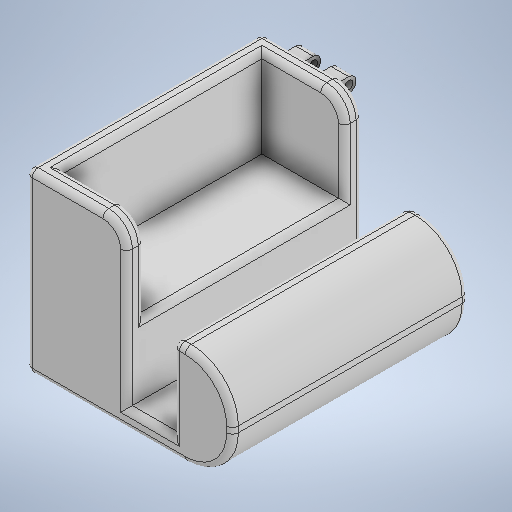
# Autodesk Inventor part: scrambler_chariot
Saved by Autodesk Inventor 2025.2 (Build 292293000, 293)
## iProperties
Created: 2025-10-10
Part Number: scrambler_chariot
Material: Generic
Document SubType Name: Modeling
Designer: pascu
Density: 1 g/cm^3
Appearance: Default
Mass: 35.9125 g
Surface Area: 129.419 cm^2
Volume: 35.9125 cm^3
Author: pascu
Autodesk Inventor part; units mm, degrees
ref_plane "YZ Plane" through (0, 0, 0) normal (1, 0, 0) x (0, 1, 0)
ref_plane "XZ Plane" through (0, 0, 0) normal (0, 1, 0) x (-1, 0, 0)
sketch "Sketch1" plane through (0, 0, 0) normal (0, 1, 0) x (-1, 0, 0)
  line L0 (0, 0) -> (-44.45, 0)
  line L1 (-44.45, 0) -> (-44.45, -50.8)
  line L2 (-44.45, -50.8) -> (0, -50.8)
  line L3 (0, -50.8) -> (0, 0)
  dimension "d0" = 44.45
  dimension "d1" = 50.8
  constraints: 8 end point, 2 parallel, 1 horizontal, 1 perpendicular
  measures "d0" distance of L2.end L1.end
  measures "d1" distance of L1.end L0.end
extrude "Extrusion1" add sketch "Sketch1" along normal blind 38.1
sketch "Sketch2" plane through (0, 38.1, 0) normal (0, 1, 0) x (1, 0, 0)
  line L0 (3.81, 3.81) -> (21.59, 3.81)
  line L1 (21.59, 3.81) -> (21.59, 46.99)
  line L2 (21.59, 46.99) -> (3.81, 46.99)
  line L3 (3.81, 46.99) -> (3.81, 3.81)
  line L4 (44.45, 50.8) -> (0, 50.8) projected
  line L5 (0, 50.8) -> (0, 0) projected
  line L6 (0, 0) -> (44.45, 0) projected
  dimension "d4" = 3.81
  dimension "d5" = 3.81
  dimension "d6" = 3.81
  dimension "d7" = 21.59
  constraints: 8 end point, 2 parallel, 1 horizontal, 1 perpendicular
  measures "d4" distance between parallel lines of L4 L2
  measures "d5" distance between parallel lines of L5 L3
  measures "d6" distance between parallel lines of L6 L0
  measures "d7" distance between parallel lines of L5 L1
extrude "Extrusion2" cut sketch "Sketch2" against normal blind 19.05
sketch "Sketch3" plane through (0, 38.1, 0) normal (0, 1, 0) x (1, 0, 0)
  line L0 (21.59, 46.99) -> (21.59, 3.81) projected
  line L1 (21.59, 0) -> (31.75, 0)
  line L2 (31.75, 0) -> (31.75, 50.8)
  line L3 (31.75, 50.8) -> (21.59, 50.8)
  line L4 (44.45, 50.8) -> (0, 50.8) projected
  line L5 (0, 0) -> (44.45, 0) projected
  line L6 (21.59, 50.8) -> (21.59, 0)
  dimension "d10" = 10.16
  constraints: 8 end point, 2 collinear, 1 horizontal, 1 parallel, 1 perpendicular, 1 vertical
  measures "d10" distance of L3.end L2.end
extrude "Extrusion3" cut sketch "Sketch3" against normal blind 34.29
sketch "Sketch4" plane through (0, 38.1, 0) normal (0, 1, 0) x (1, 0, 0)
  line L0 (44.45, 50.8) -> (31.75, 50.8) projected
  line L1 (44.45, 0) -> (44.45, 50.8) projected
  line L2 (31.75, 50.8) -> (31.75, 0) projected
  line L3 (31.75, 0) -> (44.45, 0) projected
  point P0 (0, 0)
extrude "Extrusion4" cut sketch "Sketch4" against normal blind 16.51
fillet "Fillet1" radius 10.16 2 edges at (44.45, 21.59, -25.4) (44.45, 0, -25.4)
ref_plane "Work Plane1" through (0, 0, -3.81) normal (0, 0, 1) x (1, 0, 0)
sketch "Sketch5" plane through (0, 0, -3.81) normal (0, 0, 1) x (1, 0, 0)
  arc A0 (44.45, 11.43) -> (34.29, 21.59) centre (34.29, 11.43) ccw projected
  arc A1 (34.29, 0) -> (44.45, 10.16) centre (34.29, 10.16) ccw projected
  line L0 (44.45, 10.16) -> (44.45, 11.43) projected
  arc A2 (40.64, 11.43) -> (34.29, 17.78) centre (34.29, 11.43) ccw
  line L1 (40.64, 11.43) -> (40.64, 10.16)
  arc A3 (34.29, 3.81) -> (40.64, 10.16) centre (34.29, 10.16) ccw
  line L2 (34.29, 17.78) -> (31.75, 17.78)
  line L3 (31.75, 3.81) -> (31.75, 21.59) projected
  line L4 (34.29, 3.81) -> (31.75, 3.81)
  line L5 (31.75, 3.81) -> (31.75, 17.78)
  point P0 (0, 0)
  dimension "d17" = 3.81
  constraints: 8 end point, 4 point on circle, 2 centre point, 2 horizontal, 1 collinear, 1 point on line, 2 other
  measures "d17" radial gap between concentric circles of A0 A2
extrude "Extrusion5" cut sketch "Sketch5" against normal blind 43.18
fillet "Fillet2" radius 5.08 2 edges at (21.59, 38.1, -1.905) (21.59, 38.1, -48.895)
fillet "Fillet3" radius 1.27 16 edges at (0, 38.1, -25.4) (3.81, 38.1, -25.4) (21.59, 19.05, -25.4) (0, 19.05, 0) (41.4742, 2.9758, 0) (44.45, 10.795, 0) (41.4742, 18.6142, 0) (33.02, 21.59, 0) (17.145, 0, 0) (41.4742, 18.6142, -50.8) (33.02, 21.59, -50.8) (41.4742, 2.9758, -50.8) (17.145, 0, -50.8) (44.45, 10.795, -50.8) (0, 19.05, -50.8) (0, 0, -25.4)
fillet "Fillet4" radius 1.27 18 edges at (20.1021, 36.6121, -50.8) (8.89, 38.1, -50.8) (0.372, 37.728, -50.428) (21.59, 18.415, -50.8) (20.1021, 36.6121, -46.99) (10.16, 38.1, -46.99) (3.175, 38.1, -46.99) (21.59, 18.415, -46.99) (21.59, 26.035, -46.99) (20.1021, 36.6121, -3.81) (10.16, 38.1, -3.81) (3.175, 38.1, -3.81) (21.59, 18.415, -3.81) (21.59, 26.035, -3.81) (20.1021, 36.6121, 0) (8.89, 38.1, 0) (0.372, 37.728, -0.372) (21.59, 18.415, 0)
fillet "Fillet5" radius 1.27 2 edges at (26.035, 3.81, -50.8) (26.035, 3.81, 0)
fillet "Fillet6" radius 1.27 7 edges at (31.75, 21.218, -50.428) (31.75, 21.59, -25.4) (31.75, 21.218, -0.372) (31.75, 12.065, 0) (31.75, 3.175, 0) (31.75, 12.065, -50.8) (31.75, 3.175, -50.8)
sketch "Sketch6" plane through (34.29, 1.27, -50.8) normal (0, 0, -1) x (-1, 0, 0)
  line L0 (33.02, 0) -> (0, 0) projected
  line L1 (13.9788, 0) -> (25.4088, 0)
  line L2 (25.4088, 0) -> (25.4088, 3.175)
  line L3 (25.4088, 3.175) -> (13.9788, 3.175)
  line L4 (13.9788, 3.175) -> (13.9788, 0)
  arc A0 (17.78, 35.56) -> (13.97, 31.75) centre (17.78, 31.75) ccw projected
  line L5 (17.78, 35.56) -> (29.21, 35.56)
  line L6 (29.21, 35.56) -> (29.21, 32.385)
  line L7 (29.21, 32.385) -> (17.78, 32.385)
  line L8 (17.78, 32.385) -> (17.78, 35.56)
  point P0 (34.29, -1.27)
  point P1 (25.4088, 0)
  dimension "d25" = 11.43
  dimension "d26" = 3.175
  dimension "d27" = 11.43
  dimension "d28" = 3.175
  constraints: 16 end point, 4 parallel, 2 horizontal, 2 perpendicular, 1 point on line
  measures "d25" distance of L3.end L2.end
  measures "d26" distance of L2.end L1.end
  measures "d27" distance of L6.end L7.end
  measures "d28" distance of L5.end L6.end
extrude "Extrusion6" add sketch "Sketch6" along normal blind 3.81
sketch "Sketch7" plane through (34.29, 1.27, -54.61) normal (0, 0, -1) x (-1, 0, 0)
  line L0 (29.21, 32.385) -> (17.78, 32.385) projected
  line L1 (21.59, 32.385) -> (25.4, 32.385)
  line L2 (25.4, 32.385) -> (25.4, 35.56)
  line L3 (25.4, 35.56) -> (21.59, 35.56)
  line L4 (21.59, 35.56) -> (21.59, 32.385)
  line L5 (29.21, 32.385) -> (29.21, 35.56) projected
  line L6 (17.78, 35.56) -> (17.78, 32.385) projected
  line L7 (13.9788, 3.175) -> (13.9788, 0) projected
  line L8 (13.9788, 0) -> (25.4088, 0) projected
  line L9 (17.7888, 0) -> (21.5988, 0)
  line L10 (21.5988, 0) -> (21.5988, 3.175)
  line L11 (21.5988, 3.175) -> (17.7888, 3.175)
  line L12 (17.7888, 3.175) -> (17.7888, 0)
  line L13 (25.4088, 0) -> (25.4088, 3.175) projected
  line L14 (25.4088, 3.175) -> (13.9788, 3.175) projected
  point P0 (34.29, -1.27)
  dimension "d31" = 3.175
  dimension "d32" = 3.81
  dimension "d33" = 3.81
  dimension "d34" = 3.175
  dimension "d35" = 3.81
  dimension "d36" = 3.81
  constraints: 16 end point, 4 parallel, 2 horizontal, 2 perpendicular, 1 collinear, 1 point on line
  measures "d31" distance of L1.end L2.end
  measures "d32" distance between parallel lines of L5 L2
  measures "d33" distance between parallel lines of L6 L4
  measures "d34" distance of L9.end L10.end
  measures "d35" distance between parallel lines of L7 L12
  measures "d36" distance between parallel lines of L13 L10
extrude "Extrusion7" cut sketch "Sketch7" against normal blind 3.81 contours L0 L4 L3 L2 | L11 L10 L8 L12
fillet "Fillet7" radius 1.5875 8 edges at (18.4062, 4.445, -54.61) (18.4062, 1.27, -54.61) (10.7862, 4.445, -54.61) (10.7862, 1.27, -54.61) (14.605, 33.655, -54.61) (14.605, 36.83, -54.61) (6.985, 33.655, -54.61) (6.985, 36.83, -54.61)
sketch "Sketch8" plane through (16.51, 33.655, -50.8) normal (1, 0, 0) x (0, 0, -1)
  arc A0 (2.2225, 0) -> (2.2225, 3.175) centre (2.2225, 1.5875) ccw projected
  point P0 (-50.8, -33.655)
  constraints: 1 coincident
hole "Hole1" at (16.51, 35.2425, -53.0225) direction (-1, 0, 0) diameter 1.778 end through all
sketch "Sketch9" plane through (20.3112, 1.27, -50.3303) normal (1, 0, 0) x (0, 0, -1)
  arc A0 (2.2225, 0) -> (2.2225, 3.175) centre (2.6922, 1.5875) ccw
  arc A1 (2.6922, 0) -> (2.6922, 3.175) centre (2.6922, 1.5875) ccw projected
  point P0 (-50.8, -33.655)
  constraints: 2 point on circle, 1 centre point, 1 coincident, 1 concentric
hole "Hole2" at (20.3112, 2.8575, -53.0225) direction (-1, 0, 0) diameter 1.778 end through all
body "Solid1"
